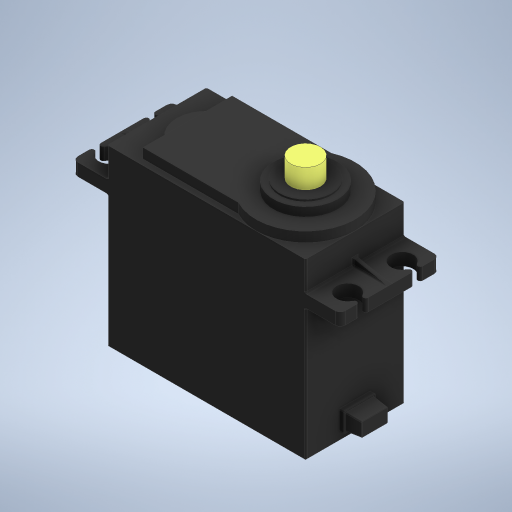
# Autodesk Inventor part: MG955서보모터
Saved by Autodesk Inventor 2023.1 (Build 271208000, 208)
## iProperties
Created: 2021-08-22
Part Number: MG955서보모터
Material: 일반
Document SubType Name: Modeling
Designer: fly01
Density: 1 g/cm^3
Appearance: 기본값
Author: fly01
Autodesk Inventor part; units mm, degrees
ref_plane "YZ Plane" through (0, 0, 0) normal (1, 0, 0) x (0, 1, 0)
ref_plane "XZ Plane" through (0, 0, 0) normal (0, 1, 0) x (-1, 0, 0)
ref_plane "XY Plane" through (0, 0, 0) normal (0, 0, 1) x (1, 0, 0)
sketch "스케치1" plane through (0, 0, 0) normal (0, 1, 0) x (-1, 0, 0)
  line L0 (20, 10) -> (-20, 10)
  line L1 (-20, 10) -> (-20, -10)
  line L2 (-20, -10) -> (20, -10)
  line L3 (20, -10) -> (20, 10)
  line L4 (20, 10) -> (-20, -10) construction
  line L5 (-20, 10) -> (20, -10) construction
  point P0 (0, 0)
  dimension "d0" = 40
  dimension "d1" = 20
  constraints: 12 end point, 2 midpoint, 2 parallel, 1 horizontal, 1 perpendicular
  measures "d0" distance of L1.end L2.end
  measures "d1" distance of L2.end L0.start
extrude "돌출1" add sketch "스케치1" along normal blind 37
ref_plane "작업 평면1" through (0, 31, 0) normal (0, 1, 0) x (1, 0, 0)
sketch "스케치2" plane through (0, 31, 0) normal (0, 1, 0) x (1, 0, 0)
  line L0 (-27, -10) -> (27, -10)
  line L1 (27, -10) -> (27, 10)
  line L2 (27, 10) -> (-27, 10)
  line L3 (-27, 10) -> (-27, -10)
  line L4 (-27, -10) -> (27, 10) construction
  line L5 (27, -10) -> (-27, 10) construction
  point P0 (0, 0)
  point P1 (-20, 10)
  dimension "d5" = 54
  constraints: 12 end point, 2 midpoint, 2 parallel, 1 horizontal, 1 perpendicular, 1 point on line
  measures "d5" distance of L1.end L2.end
extrude "돌출2" add sketch "스케치2" against normal blind 2.5
sketch "스케치3" plane through (0, 31, 0) normal (0, 1, 0) x (1, 0, 0)
  arc A0 (-26.1937, 5) -> (-26.1937, 6) centre (-24, 5.5) ccw
  line L0 (-20, 10) -> (-27, 10) projected
  line L1 (-27.6923, 6) -> (-26.1937, 6)
  line L2 (-26.1937, 5) -> (-27.6923, 5)
  line L3 (-27.6923, 5) -> (-27.6923, 6)
  line L4 (-27.6923, 6) -> (-24.8077, 5) construction
  line L5 (-24.8077, 6) -> (-27.6923, 5) construction
  line L6 (-27, 10) -> (-27, -10) projected
  line L7 (0, 0) -> (0, 3.5)
  line L8 (0, 0) -> (-2.0825, 0)
  arc A1 (26.1937, 6) -> (26.1937, 5) centre (24, 5.5) ccw
  line L9 (27.6923, 6) -> (26.1937, 6)
  line L10 (26.1937, 5) -> (27.6923, 5)
  line L11 (27.6923, 5) -> (27.6923, 6)
  arc A2 (-26.1937, -6) -> (-26.1937, -5) centre (-24, -5.5) ccw
  line L12 (-27.6923, -6) -> (-26.1937, -6)
  line L13 (-26.1937, -5) -> (-27.6923, -5)
  line L14 (-27.6923, -5) -> (-27.6923, -6)
  line L15 (26.1937, -5) -> (27.6923, -5)
  line L16 (27.6923, -5) -> (27.6923, -6)
  arc A3 (26.1937, -5) -> (26.1937, -6) centre (24, -5.5) ccw
  line L17 (27.6923, -6) -> (26.1937, -6)
  dimension "d8" = 4.5
  dimension "d9" = 4.5
  dimension "d10" = 3
  dimension "d11" = 1
  constraints: 32 end point, 15 symmetric about line, 8 point on circle, 4 centre point, 2 horizontal, 1 parallel, 1 vertical, 3 other
  measures "d8" distance from line of L0 A0.centre
  measures "d9" diameter of A0
  measures "d10" distance from line of L6 A0.centre
  measures "d11" distance of L2.end L1.start
extrude "돌출3" cut sketch "스케치3" against normal blind 4.5
sketch "스케치4" plane through (0, 0, 0) normal (0, 0, 1) x (1, 0, 0)
  line L0 (-27, 31) -> (-20, 31) projected
  line L1 (-27, 31) -> (-20, 32.4)
  line L2 (-20, 31) -> (-20, 37) projected
  point P0 (0, 0)
  dimension "d14" = 1.4
  constraints: 2 end point, 1 point on line
  measures "d14" distance of L0.end L1.end
extrude "돌출4" add sketch "스케치4" along normal mid plane 0.7
mirror "미러1" about plane through (0, 0, 0) normal (1, 0, 0) of "돌출4"
sketch "스케치5" plane through (0, 37, 0) normal (0, 1, 0) x (1, 0, 0)
  line L0 (20, -10) -> (20, 10) projected
  line L1 (20, 0) -> (10, 0)
  circle A0 centre (10, 0) radius 10
  line L2 (-14, 9.1754) -> (6.0235, 9.1754)
  line L3 (8.986, 9.1754) -> (8.986, -8.8246) construction
  line L4 (8.986, -8.8246) -> (5.2962, -8.8246) construction
  line L5 (-14, -8.8246) -> (-14, 9.1754)
  line L6 (-14, 9.1754) -> (8.986, -8.8246) construction
  line L7 (8.986, 9.1754) -> (-14, -8.8246) construction
  line L8 (-20, 10) -> (-20, -10) projected
  line L9 (5.2962, -8.8246) -> (-14, -8.8246)
  line L10 (6.0235, 9.1754) -> (8.986, 9.1754) construction
  point P0 (0, 0)
  point P1 (-2.507, 0.1754)
  dimension "d17" = 10
  dimension "d18" = 20
  dimension "d19" = 18
  dimension "d20" = 6
  constraints: 18 end point, 5 parallel, 3 horizontal, 3 midpoint, 2 perpendicular, 2 point on circle, 1 centre point, 1 coincident
  measures "d17" distance of L1.start L1.end
  measures "d18" diameter of A0
  measures "d19" distance of L3.start L3.end
  measures "d20" distance between parallel lines of L8 L5
extrude "돌출5" add sketch "스케치5" along normal blind 2
sketch "스케치6" plane through (0, 37, 0) normal (0, 1, 0) x (1, 0, 0)
  line L0 (-14, -8.8246) -> (-14, 9.1754) projected
  line L1 (-14, 0) -> (-16, 0)
  line L2 (-14, 0) -> (-14, 4.5)
  line L3 (-14, 4.5) -> (-14, -4.5)
  arc A0 (-14, 4.5) -> (-14, -4.5) centre (-9.9375, 0) ccw
  point P0 (0, 0)
  dimension "d23" = 2
  dimension "d24" = 4.5
  dimension "d25" = 9
  constraints: 6 end point, 3 point on circle, 3 point on line, 1 centre point, 1 horizontal
  measures "d23" distance of L1.start L1.end
  measures "d24" distance of L1.start L2.end
  measures "d25" distance of L2.end L3.end
extrude "돌출6" add sketch "스케치6" along normal blind 1.7
sketch "스케치7" plane through (0, 39, 0) normal (0, 1, 0) x (1, 0, 0)
  arc A0 (5.2962, -8.8246) -> (6.0235, 9.1754) centre (10, 0) ccw projected
  circle A1 centre (10, 0) radius 6.5
  circle A2 centre (10, 0) radius 5.25
  point P0 (0, 0)
  dimension "d28" = 13
  dimension "d29" = 10.5
  constraints: 2 centre point, 2 coincident
  measures "d28" diameter of A1
  measures "d29" diameter of A2
extrude "돌출7" add sketch "스케치7" along normal blind 1.8 contours A1 | A2
extrude "돌출8" add sketch "스케치7" along normal blind 2.2 contours A2
sketch "스케치8" plane through (10, 41.2, 0) normal (0, 1, 0) x (1, 0, 0)
  circle A0 centre (0, 0) radius 5.25 projected
  circle A1 centre (0, 0) radius 3
  point P0 (-10, 0)
  dimension "d34" = 6
  constraints: 1 centre point, 1 coincident
  measures "d34" diameter of A1
extrude "돌출9" add sketch "스케치8" along normal blind 4 contours A1
fillet "모깎기1" radius 0.5 16 edges at (-26.1937, 29.75, -6) (-27, 29.75, -6) (-26.1937, 29.75, 5) (-27, 29.75, 5) (-27, 29.75, -5) (-26.1937, 29.75, -5) (-27, 29.75, 6) (-26.1937, 29.75, 6) (26.1937, 29.75, -5) (27, 29.75, -5) (26.1937, 29.75, 6) (27, 29.75, 6) (26.1937, 29.75, -6) (27, 29.75, -6) (26.1937, 29.75, 5) (27, 29.75, 5)
fillet "모깎기2" radius 1 4 edges at (-27, 29.75, 10) (27, 29.75, 10) (27, 29.75, -10) (-27, 29.75, -10)
chamfer "모따기1" distance 2 angle 45 4 edges at (20, 0, 0) (-20, 0, 0) (0, 0, 10) (0, 0, -10)
fillet "모깎기3" radius 0.3 8 edges at (-20, 15.25, 10) (-20, 34, 10) (20, 34, 10) (20, 15.25, 10) (-20, 34, -10) (-20, 15.25, -10) (20, 15.25, -10) (20, 34, -10)
fillet "모깎기4" radius 0.3 18 edges at (19.9121, 31, -9.9121) (20, 31, -5.025) (23.5, 31, -0.35) (23.5, 31, 0.35) (19.9121, 31, 9.9121) (20, 31, 5.025) (-19.9121, 31, 9.9121) (-20, 31, 5.025) (-19.9121, 31, -9.9121) (-20, 31, -5.025) (-23.5, 31, -0.35) (-23.5, 31, 0.35) (-20, 31.7, 0.35) (-20, 31.7, -0.35) (-20, 32.4, 0) (20, 31.7, -0.35) (20, 32.4, 0) (20, 31.7, 0.35)
fillet "모깎기5" radius 0.3 6 edges at (-19.9121, 28.5, -9.9121) (-19.9121, 28.5, 9.9121) (-20, 28.5, 0) (19.9121, 28.5, 9.9121) (19.9121, 28.5, -9.9121) (20, 28.5, 0)
sketch "스케치9" plane through (20, 2, 9.7) normal (1, 0, 0) x (0, 0, -1)
  line L0 (9.7, -2) -> (9.7, 5.5)
  line L1 (6.5, 5.5) -> (12.9, 5.5)
  line L2 (12.9, 5.5) -> (12.9, 1.5)
  line L3 (12.9, 1.5) -> (6.5, 1.5)
  line L4 (6.5, 1.5) -> (6.5, 5.5)
  line L5 (6.5, 5.5) -> (12.9, 1.5) construction
  line L6 (12.9, 5.5) -> (6.5, 1.5) construction
  point P0 (9.7, 3.5)
  dimension "d45" = 7.5
  dimension "d46" = 4
  dimension "d47" = 6.4
  constraints: 14 end point, 3 midpoint, 2 parallel, 1 horizontal, 1 perpendicular, 1 point on line, 1 vertical
  measures "d45" distance of L0.start L0.end
  measures "d46" distance of L1.end L2.end
  measures "d47" distance of L1.start L1.end
extrude "돌출10" add sketch "스케치9" along normal blind 1
sketch "스케치10" plane through (21, 2, 9.7) normal (1, 0, 0) x (0, 0, -1)
  line L0 (6.5, 1.5) -> (12.9, 1.5) projected
  line L1 (12.9, 1.5) -> (12.9, 5.5) projected
  line L2 (12.9, 5.5) -> (6.5, 5.5) projected
  line L3 (6.5, 5.5) -> (6.5, 1.5) projected
  line L4 (6.8, 5.2) -> (12.6, 5.2)
  line L5 (12.6, 5.2) -> (12.6, 1.8)
  line L6 (12.6, 1.8) -> (6.8, 1.8)
  line L7 (6.8, 1.8) -> (6.8, 5.2)
  point P0 (9.7, -2)
  dimension "d50" = 0.3
  constraints: 8 end point, 3 other
  measures "d50" distance between parallel lines of L2 L4
extrude "돌출11" add sketch "스케치10" along normal blind 3 contours L4 L5 L6 L7
chamfer "모따기2" distance 3 angle 5 1 edges at (24, 3.8, 0) measured on face at (23.5, 3.8, 0)
chamfer "모따기3" distance 3 angle 5 1 edges at (24, 5.6312, -2.9) measured on face at (23.5, 5.6312, -2.9)
chamfer "모따기4" distance 3 angle 5 1 edges at (24, 7.2, 0.1312) measured on face at (23.5, 7.2, 0.1312)
chamfer "모따기5" distance 3 angle 5 1 edges at (24, 5.5, 2.9) measured on face at (23.5, 5.5, 2.9)
fillet "모깎기6" radius 0.2 14 edges at (20.5, 7.5, 3.2) (20.5, 3.5, 3.2) (20.5, 7.5, -3.2) (20.5, 3.5, -3.2) (22.5006, 7.0688, -2.7688) (21.0006, 7.2, -2.9) (22.5006, 3.9313, -2.7688) (21.0006, 3.8, -2.9) (21.0001, 3.8, -2.9) (22.5006, 7.0688, 2.7688) (21.0006, 7.2, 2.9) (22.5006, 3.9313, 2.7688) (21.0006, 3.8, 2.9) (21.0001, 3.8, 2.9)
fillet "모깎기7" radius 0.1 16 edges at (24, 6.8794, 2.5794) (24, 6.9376, 0) (24, 6.8794, -2.5794) (24, 5.5, -2.6376) (24, 4.1207, -2.5794) (24, 4.0625, 0) (24, 4.1207, 2.5794) (24, 5.5, 2.6376) (21, 3.5586, 3.1414) (21, 3.5, 0) (21, 3.5586, -3.1414) (21, 5.5, -3.2) (21, 7.4414, -3.1414) (21, 7.5, 0) (21, 7.4414, 3.1414) (21, 5.5, 3.2)
sketch "스케치13" plane through (0, 39, 0) normal (0, 1, 0) x (1, 0, 0)
  line L0 (-20, 9.7) -> (-20, -9.7) projected
  line L1 (20, -9.7) -> (20, 0) projected
  arc A0 (-26.0455, -6.4373) -> (-26.0455, -4.5627) centre (-24, -5.5) ccw projected
  arc A1 (26.0455, -4.5627) -> (26.0455, -6.4373) centre (24, -5.5) ccw projected
  line L2 (-27, -6.6456) -> (-27, -9) projected
  line L3 (27, -9) -> (27, -6.6456) projected
  line L4 (20.2196, -10) -> (26, -10) projected
  line L5 (26, 10) -> (20.2196, 10) projected
  point P0 (0, 0)
  dimension "d67" = 40
  dimension "d68" = 48
  dimension "d69" = 54
  dimension "d70" = 20
  measures "d67" distance between parallel lines of L0 L1
  measures "d68" distance of A0.centre A1.centre
  measures "d69" distance between parallel lines of L2 L3
  measures "d70" distance between parallel lines of L4 L5
sketch "스케치14" plane through (10, 45.2, 0) normal (0, 1, 0) x (1, 0, 0)
  arc A0 (16.0455, -4.5627) -> (16.0455, -6.4373) centre (14, -5.5) ccw projected
  arc A1 (16.0455, 6.4373) -> (16.0455, 4.5627) centre (14, 5.5) ccw projected
  point P0 (-10, 0)
  dimension "d71" = 11
  measures "d71" distance of A0.centre A1.centre
equation "\"d12\" = d8"
